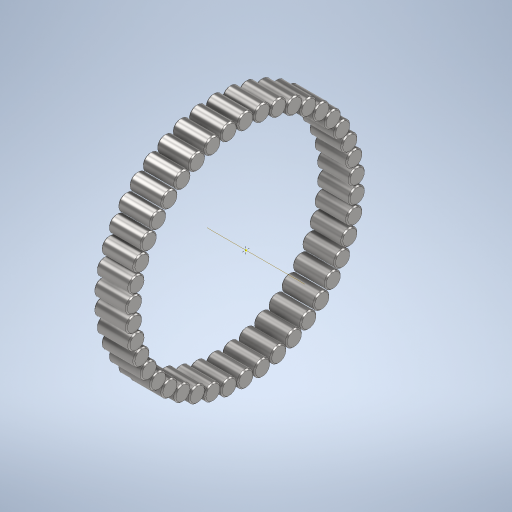
# Autodesk Inventor part: bearing_stifts_antenna
Saved by Autodesk Inventor 2024 (Build 280153000, 153)
## iProperties
Created: 2025-12-27
Part Number: bearing_stifts_antenna
Material: Stainless Steel
Document SubType Name: Modeling
Designer: schar
Density: 8 g/cm^3
Appearance: Semi-Polished
Author: schar
Autodesk Inventor part; units mm, degrees
ref_plane "YZ Plane" through (0, 0, 0) normal (1, 0, 0) x (0, 1, 0)
ref_plane "XZ Plane" through (0, 0, 0) normal (0, 1, 0) x (-1, 0, 0)
ref_plane "XY Plane" through (0, 0, 0) normal (0, 0, 1) x (1, 0, 0)
sketch "Sketch3" plane through (0, 0, 0) normal (1, 0, 0) x (0, 1, 0)
  circle A0 centre (0, 0) radius 20.5
  circle A1 centre (20.5, 0) radius 1.5
  dimension "d5" = 41
  dimension "d6" = 3
  constraints: 1 centre point, 1 coincident, 1 horizontal alignment, 2 other
  measures "d6" diameter of A1
extrude "Extrusion2" add sketch "Sketch3" along normal blind 6 contours A0 A1 | A0 A1 picked at (20.029, 0.34) picked at (20.9462, 0.3883)
chamfer "Chamfer1" distance 0.2 angle 45 2 edges at (6, 19, 0) (0, 19, 0)
pattern_circular "Circular Pattern1" count 42 over 360 about axis through (-10, 0, 0) along (1, 0, 0) of "Extrusion2", "Chamfer1"
sketch "Sketch4" plane through (6, 12.7815, 16.0275) normal (1, 0, 0) x (0, 0, -1)
  point P0 (16.0275, -12.7815)
  point P1 (16.0275, -12.7815)
  constraints: 1 coincident
body "Solid2"
